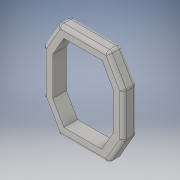
# Autodesk Inventor part: Bumpers
Saved by Autodesk Inventor 2016 (Build 200138000, 138)
## iProperties
Created: 2016-02-01
Part Number: Bumpers
Material: Generic
Document SubType Name: Modeling
Designer: Mentor1102
Density: 1 g/cm^3
Appearance: Default
Author: Mentor1102
Autodesk Inventor part; units mm, degrees
ref_plane "YZ Plane" through (0, 0, 0) normal (1, 0, 0) x (0, 1, 0)
ref_plane "XZ Plane" through (0, 0, 0) normal (0, 1, 0) x (-1, 0, 0)
ref_plane "XY Plane" through (0, 0, 0) normal (0, 0, 1) x (1, 0, 0)
sketch "Sketch1" plane through (0, 0, 0) normal (0, 0, 1) x (1, 0, 0)
  line L0 (0, 0) -> (351.6706, 0)
  line L1 (-103.5647, 179.3793) -> (0, 0)
  line L2 (351.6706, 0) -> (455.2353, 179.3793)
  line L3 (455.2353, 179.3793) -> (455.2353, 534.9793)
  line L4 (-103.5647, 534.9793) -> (-103.5647, 179.3793)
  line L5 (0, 714.3586) -> (-103.5647, 534.9793)
  line L6 (356.3091, 714.3586) -> (0, 714.3586)
  line L7 (455.2353, 534.9793) -> (356.3091, 714.3586)
  line L8 (-103.5647, 179.3793) -> (-192.4647, 179.3793) construction
  line L9 (-51.7823, 89.6897) -> (-128.772, 45.2397) construction
  line L10 (-128.772, 45.2397) -> (-51.7823, -88.9)
  line L11 (-51.7823, -88.9) -> (0, -88.9)
  line L12 (178.1545, -88.9) -> (178.1545, 714.3586) construction
  line L13 (178.1545, -88.9) -> (0, -88.9)
  line L14 (-128.772, 45.2397) -> (-192.4647, 156.2119)
  line L15 (-192.4647, 156.2119) -> (-192.4647, 179.3793)
  line L16 (178.1545, 714.3586) -> (178.1545, 803.2586) construction
  line L17 (-51.7823, 624.669) -> (-128.772, 669.119) construction
  line L18 (-192.4647, 179.3793) -> (-192.4647, 558.8)
  line L19 (-192.4647, 558.8) -> (-128.772, 669.119)
  line L20 (178.1545, 803.2586) -> (-51.3264, 803.2586)
  line L21 (-51.3264, 803.2586) -> (-128.772, 669.119)
  line L22 (485.0811, 45.2397) -> (408.0914, -88.9)
  line L23 (178.1545, -88.9) -> (356.3091, -88.9)
  line L24 (485.0811, 45.2397) -> (548.7738, 156.2119)
  line L25 (548.7738, 156.2119) -> (548.7738, 179.3793)
  line L26 (408.0914, 624.669) -> (485.0811, 669.119) construction
  line L27 (548.7738, 179.3793) -> (548.7738, 558.8)
  line L28 (548.7738, 558.8) -> (485.0811, 669.119)
  line L29 (178.1545, 803.2586) -> (407.6355, 803.2586)
  line L30 (407.6355, 803.2586) -> (485.0811, 669.119)
  line L31 (408.0914, -88.9) -> (356.3091, -88.9)
  point P0 (175.8353, 357.1793)
  dimension "d0" = 88.9
  dimension "d1" = 88.9
  dimension "d2" = 88.9
  dimension "d3" = 88.9
  dimension "d4" = 88.9
  dimension "d8" = 88.9
  constraints: 64 end point, 10 symmetric about line, 4 point on line, 3 horizontal, 3 midpoint, 3 perpendicular, 2 collinear, 2 vertical
  measures "d0" distance of L0.start L11.end
  measures "d1" distance of L1.start L8.end
  measures "d2" distance of L9.start L9.end
  measures "d3" distance of L12.end L16.end
  measures "d4" distance of L17.start L17.end
  measures "d8" distance between parallel lines of L18 L4
extrude "Extrusion1" add sketch "Sketch1" along normal blind 127
fillet "Fillet1" radius 31.75 24 edges at (63.414, 803.2586, 127) (446.3583, 736.1888, 127) (548.7738, 369.0897, 127) (516.9274, 100.7258, 127) (89.0773, -88.9, 127) (-90.2772, -21.8302, 127) (-192.4647, 167.7956, 127) (-160.6184, 613.9595, 127) (548.7738, 369.0897, 0) (516.9274, 613.9595, 0) (63.414, 803.2586, 0) (-160.6184, 613.9595, 0) (-192.4647, 167.7956, 0) (-90.2772, -21.8302, 0) (-25.8912, -88.9, 0) (446.5863, -21.8302, 0) (548.7738, 156.2119, 63.5) (548.7738, 558.8, 63.5) (407.6355, 803.2586, 63.5) (-51.3264, 803.2586, 63.5) (-192.4647, 558.8, 63.5) (-192.4647, 156.2119, 63.5) (-51.7823, -88.9, 63.5) (408.0914, -88.9, 63.5)
body "Solid1"
